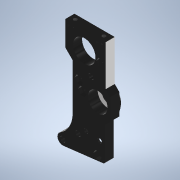
# Autodesk Inventor part: PartB_3gears_3D
Saved by Autodesk Inventor 2022 (Build 260153000, 153)
## iProperties
Created: 2020-12-02
Part Number: PartB_3gears_3D
Material: Generic
Document SubType Name: Modeling
Designer: Acer
Density: 1 g/cm^3
Appearance: Default
Author: Acer
Autodesk Inventor part; units mm, degrees
ref_plane "YZ Plane" through (0, 0, 0) normal (1, 0, 0) x (0, 1, 0)
ref_plane "XZ Plane" through (0, 0, 0) normal (0, 1, 0) x (-1, 0, 0)
ref_plane "XY Plane" through (0, 0, 0) normal (0, 0, 1) x (1, 0, 0)
sketch "Sketch1" plane through (0, 0, 0) normal (0, 0, 1) x (1, 0, 0)
  circle A0 centre (0, 0) radius 1.5
  circle A1 centre (0, 0) radius 3
  line L0 (0, 3) -> (23.5, 3)
  line L1 (23.5, 3) -> (23.5, -3)
  line L2 (23.5, -3) -> (0, -3)
  line L3 (0, -3) -> (0, 3)
  line L4 (23.5, 3) -> (5.5, 3)
  line L5 (5.5, 3) -> (5.5, 59)
  line L6 (5.5, 59) -> (23.5, 59)
  line L7 (23.5, 59) -> (23.5, 3)
  circle A2 centre (19.5, 27.75) radius 5.5
  circle A3 centre (11.9973, 48.75) radius 6.25
  line L8 (19.5, 27.75) -> (11.9973, 48.75) construction
  line L9 (19.5, 27.75) -> (5.5, 27.75) construction
  circle A4 centre (11.9973, 40.25) radius 1.05
  circle A5 centre (19.3585, 53) radius 1.05
  circle A6 centre (4.6361, 53) radius 1.05
  line L10 (5.5, 59) -> (1.5, 59)
  line L11 (1.5, 59) -> (1.5, 45)
  line L12 (1.5, 45) -> (5.5, 45)
  line L13 (5.5, 45) -> (5.5, 59)
  line L14 (1.5, 45) -> (5.5, 41)
  line L15 (1.5, 45) -> (7.1569, 45) construction
  line L16 (23.5, 33.75) -> (26.5, 33.75)
  line L17 (26.5, 33.75) -> (26.5, 21.75)
  line L18 (26.5, 21.75) -> (23.5, 21.75)
  line L19 (23.5, 21.75) -> (23.5, 33.75)
  line L20 (26.5, 33.75) -> (23.5, 36.75)
  line L21 (26.5, 33.75) -> (30.7426, 33.75) construction
  line L22 (26.5, 21.75) -> (23.5, 18.75)
  line L23 (26.5, 21.75) -> (30.7426, 21.75) construction
  circle A7 centre (8.5, 7) radius 1.5
  circle A8 centre (13, 10.5) radius 1.25
  circle A9 centre (20.5, 9.5) radius 1.25
  line L24 (11.9973, 48.75) -> (1.5, 48.75) construction
  line L25 (11.9973, 40.25) -> (11.9973, 48.75) construction
  circle A10 centre (15.7487, 38.25) radius 1.55
  circle A11 centre (11, 28.75) radius 1.05
  circle A12 centre (9, 33.25) radius 1.05
  circle A13 centre (21, 47.25) radius 1.05
  line L26 (5.5, 27) -> (23.5, 27) construction
  line L27 (23.5, 27) -> (23.5, 51) construction
  line L28 (23.5, 51) -> (5.5, 51) construction
  line L29 (5.5, 51) -> (5.5, 27) construction
  line L30 (7.7876, 31.15) -> (6.5751, 33.25) construction
  line L31 (6.5751, 33.25) -> (7.7876, 35.35) construction
  line L32 (7.7876, 35.35) -> (10.2124, 35.35) construction
  line L33 (10.2124, 35.35) -> (11.4249, 33.25) construction
  line L34 (11.4249, 33.25) -> (10.2124, 31.15) construction
  line L35 (10.2124, 31.15) -> (7.7876, 31.15) construction
  line L36 (9.7876, 26.65) -> (8.5751, 28.75) construction
  line L37 (8.5751, 28.75) -> (9.7876, 30.85) construction
  line L38 (9.7876, 30.85) -> (12.2124, 30.85) construction
  line L39 (12.2124, 30.85) -> (13.4249, 28.75) construction
  line L40 (13.4249, 28.75) -> (12.2124, 26.65) construction
  line L41 (12.2124, 26.65) -> (9.7876, 26.65) construction
  line L42 (23.5, -0.2) -> (0.1795, -3)
  dimension "d0" = 3
  dimension "d1" = 6
  dimension "d2" = 23.5
  dimension "d3" = 6
  dimension "d4" = 0
  dimension "d5" = 3
  dimension "d6" = 18
  dimension "d7" = 56
  dimension "d8" = 11
  dimension "d9" = 4
  dimension "d10" = 24.75
  dimension "d11" = 12.5
  dimension "d12" = 22.3
  dimension "d14" = 2.1
  dimension "d20" = 360
  dimension "d22" = 4
  dimension "d23" = 14
  dimension "d24" = 45
  dimension "d25" = 3
  dimension "d26" = 12
  dimension "d27" = 6
  dimension "d28" = 135
  dimension "d29" = 135
  dimension "d32" = 3
  dimension "d33" = 10
  dimension "d34" = 3
  dimension "d35" = 2.5
  dimension "d36" = 13.5
  dimension "d37" = 7.5
  dimension "d38" = 2.5
  dimension "d39" = 15
  dimension "d40" = 12.5
  dimension "d60" = 8.5
  dimension "d61" = 270
  dimension "d82" = 3.1
  dimension "d83" = 11.15
  dimension "d84" = 2.1
  dimension "d85" = 2.1
  dimension "d86" = 2.1
  dimension "d87" = 5.5
  dimension "d88" = 3.5
  dimension "d89" = 25.75
  dimension "d90" = 30.25
  dimension "d91" = 2.5
  dimension "d92" = 11.75
  dimension "d93" = 24
  dimension "d94" = 8
  dimension "d101" = 2.1
  dimension "d102" = 2.1
  dimension "d157" = 2.8
  constraints: 86 end point, 14 centre point, 11 horizontal, 10 parallel, 10 point on line, 6 perpendicular, 4 coincident, 3 equal length, 1 midpoint, 1 tangent, 33 other
  measures "d0" diameter of A0
  measures "d1" diameter of A1
  measures "d2" distance of L1.end L2.end
  measures "d3" distance of L0.end L1.end
  measures "d4" distance from line of point (0, 0) L3
  measures "d5" distance from line of L0 point (0, 0)
  measures "d6" distance of L5.end L6.end
  measures "d7" distance of L4.end L5.end
  measures "d8" diameter of A2
  measures "d9" distance from line of L7 L8.start
  measures "d10" distance from line of L8.start L0
  measures "d11" diameter of A3
  measures "d12" distance of L8.start L8.end
  measures "d14" diameter of A4
  measures "d22" distance of L12.end L11.end
  measures "d23" distance of L11.end L10.end
  measures "d24" angle of L14 L15
  measures "d25" distance of L17.end L18.end
  measures "d26" distance of L16.end L17.end
  measures "d27" distance from line of L16 L8.start
  measures "d28" angle of L21 L20
  measures "d29" angle of L22 L23
  measures "d32" diameter of A7
  measures "d33" distance from line of L2 A7.centre
  measures "d34" distance from line of L5 A7.centre
  measures "d35" diameter of A8
  measures "d36" distance from line of A8.centre L2
  measures "d37" distance from line of L5 A8.centre
  measures "d38" diameter of A9
  measures "d39" distance from line of A9.centre L5
  measures "d40" distance from line of L2 A9.centre
  measures "d60" distance of L25.start L8.end
  measures "d82" diameter of A10
  measures "d83" distance of A10.centre L8.start
  measures "d84" diameter of A11
  measures "d85" diameter of A12
  measures "d86" diameter of A13
  measures "d87" distance from line of L5 A11.centre
  measures "d88" distance from line of L5 A12.centre
  measures "d89" distance from line of L6 A12.centre
  measures "d90" distance from line of L6 A11.centre
  measures "d91" distance from line of L7 A13.centre
  measures "d92" distance from line of L6 A13.centre
  measures "d93" distance between parallel lines of L28 L26
  measures "d94" distance between parallel lines of L6 L28
  measures "d101" distance from line of A12.centre L35
  measures "d102" distance from line of A11.centre L41
  measures "d157" distance from line of L2 L42.start
extrude "Extrusion1" add sketch "Sketch1" along normal blind 5 contours A0 L3 A1 | A0 L3 A1 | L0 L1 L42 A1 | A1 L42 L2 | L5 A6 L6 L7 A2 L0 | L14 L12 L5 | L7 L18 L22 | L12 L11 L10 L5 A6 | L7 A2 L16 L17 L18 | A6 L5 | L5 A6 | L16 L7 L20 | A4 | A5
fillet "Fillet1" radius 1 1 edges at (23.5, -0.2, 2.5)
fillet "Fillet2" radius 15 1 edges at (5.5, 3, 2.5)
sketch "Sketch2" plane through (0, 0, 5) normal (0, 0, 1) x (1, 0, 0)
  line L0 (23.5, 0.6871) -> (23.5, 18.75) projected
  line L1 (0, -3) -> (0.1795, -3) projected
  line L2 (23.5, 0.6871) -> (23.5, 18.75) projected
  line L3 (23.5, 20.75) -> (10.75, 20.75)
  line L4 (10.75, 20.75) -> (10.75, 0.75)
  line L5 (10.75, 0.75) -> (23.5, 0.75)
  line L6 (23.5, 0.75) -> (23.5, 20.75)
  line L7 (23.5, 18.75) -> (26.5, 21.75) projected
  line L8 (23.5, 20.75) -> (25.5, 20.75)
  line L9 (23.5, 18.75) -> (26.5, 21.75) projected
  line L10 (22.25, 20.75) -> (22.25, 0.75)
  point P0 (0, 0)
  point P1 (23.5, -1)
  point P2 (21.5, -3)
  point P3 (23.5, 0.75)
  point P4 (23.5, 0.5)
  point P5 (23.5, 0.75)
  dimension "d43" = 12.75
  dimension "d44" = 20
  dimension "d45" = 23.75
  constraints: 12 end point, 4 point on line, 2 horizontal, 2 parallel, 2 perpendicular
  measures "d43" distance of L5.end L4.end
  measures "d44" distance of L4.end L3.end
  measures "d45" distance between parallel lines of L1 L3
extrude "Extrusion2" [suppressed]
sketch "Sketch3" plane through (1.5, 59, 0) normal (0, 1, 0) x (1, 0, 0)
  circle A0 centre (3, -2.5) radius 1
  line L0 (22, 0) -> (0, 0) projected
  line L1 (0, 0) -> (0, -5) projected
  line L2 (22, -5) -> (0, -5) projected
  line L3 (22, 0) -> (22, -5) projected
  circle A1 centre (19, -2.5) radius 1
  dimension "d48" = 2
  dimension "d49" = 2
  dimension "d50" = 2.5
  dimension "d51" = 2.5
  dimension "d52" = 3
  dimension "d53" = 3
  constraints: 2 centre point
  measures "d48" diameter of A0
  measures "d49" diameter of A1
  measures "d50" distance from line of L0 A0.centre
  measures "d51" distance from line of L0 A1.centre
  measures "d52" distance from line of A1.centre L3
  measures "d53" distance from line of L1 A0.centre
extrude "Extrusion3" cut sketch "Sketch3" against normal blind 4.5 contours A0 | A1
thread "Thread1" size "M2x0.4" class "6H" standard "ANSI Metric M Profile" length 7
thread "Thread2" size "M2x0.4" class "6H" standard "ANSI Metric M Profile" length 7
sketch "Sketch5" plane through (0, 0, 5) normal (0, 0, 1) x (1, 0, 0)
  circle A0 centre (11.9973, 40.25) radius 1.05 projected
  circle A1 centre (4.6361, 53) radius 1.05 projected
  circle A2 centre (19.3585, 53) radius 1.05 projected
  circle A3 centre (11.9973, 40.25) radius 2
  circle A4 centre (4.6361, 53) radius 2
  circle A5 centre (19.3585, 53) radius 2
  point P0 (0, 0)
  dimension "d62" = 4
  dimension "d63" = 4
  dimension "d64" = 4
  constraints: 3 centre point, 3 coincident
  measures "d62" diameter of A3
  measures "d63" diameter of A4
  measures "d64" diameter of A5
extrude "Extrusion4" [suppressed]
sketch "Sketch7" plane through (0, 0, 5) normal (0, 0, 1) x (1, 0, 0)
  circle A0 centre (8.5, 7) radius 1.5 projected
  circle A1 centre (8.5, 7) radius 2.75
  point P0 (0, 0)
  dimension "d67" = 5.5
  constraints: 1 centre point, 1 coincident
  measures "d67" diameter of A1
extrude "Extrusion5" cut sketch "Sketch7" against normal blind 2 contours A0 | A1
sketch "Sketch8" plane through (0, 0, 5) normal (0, 0, 1) x (1, 0, 0)
  line L0 (5.5, 59) -> (5.5, 54.5) projected
  line L1 (3.5, 59) -> (3.5, 54.5) projected
  circle A0 centre (19.5, 27.75) radius 5.5 projected
  circle A1 centre (11.9973, 48.75) radius 6.25 projected
  circle A2 centre (8.5, 7) radius 2.75 projected
  line L2 (23.5, 18.75) -> (26.5, 21.75) projected
  line L3 (26.5, 21.75) -> (26.5, 33.75) projected
  line L4 (26.5, 33.75) -> (23.5, 36.75) projected
  line L5 (23.5, 36.75) -> (23.5, 59) projected
  line L6 (23.5, 59) -> (1.5, 59) projected
  line L7 (1.5, 59) -> (1.5, 45) projected
  line L8 (1.5, 45) -> (5.5, 41) projected
  line L9 (5.5, 41) -> (5.5, 15.2889) projected
  line L10 (19.5, 59) -> (19.5, 54.5) projected
  line L11 (21.5, 59) -> (21.5, 54.5) projected
  line L12 (2.5, 55.275) -> (6.5, 55.275)
  line L13 (6.5, 55.275) -> (6.5, 57.125)
  line L14 (6.5, 57.125) -> (2.5, 57.125)
  line L15 (2.5, 57.125) -> (2.5, 55.275)
  line L16 (2.5, 55.275) -> (6.5, 57.125) construction
  line L17 (6.5, 55.275) -> (2.5, 57.125) construction
  line L18 (18.5, 57.125) -> (22.5, 57.125)
  line L19 (22.5, 57.125) -> (22.5, 55.275)
  line L20 (22.5, 55.275) -> (18.5, 55.275)
  line L21 (18.5, 55.275) -> (18.5, 57.125)
  line L22 (18.5, 57.125) -> (22.5, 55.275) construction
  line L23 (22.5, 57.125) -> (18.5, 55.275) construction
  arc A3 (-1.5833, 2.5481) -> (5.5, 15.2889) centre (-9.5, 15.2889) ccw projected
  arc A4 (-1.5833, 2.5481) -> (0, -3) centre (0, 0) ccw projected
  line L24 (0, -3) -> (0.1795, -3) projected
  line L25 (23.5, 0.6871) -> (23.5, 18.75) projected
  line L26 (0.1795, -3) -> (22.6192, -0.3058) projected
  arc A5 (22.6192, -0.3058) -> (23.5, 0.6871) centre (22.5, 0.6871) ccw projected
  point P0 (4.5, 56.2)
  point P1 (20.5, 56.2)
  dimension "d70" = 4
  dimension "d71" = 1.85
  dimension "d72" = 4
  dimension "d73" = 1.85
  dimension "d74" = 1
  dimension "d75" = 2.8
  dimension "d76" = 2.8
  dimension "d77" = 1
  constraints: 24 end point, 4 midpoint, 4 parallel, 2 horizontal, 2 perpendicular
  measures "d70" distance of L14.end L13.end
  measures "d71" distance of L13.end L12.end
  measures "d72" distance of L19.end L20.end
  measures "d73" distance of L18.end L19.end
  measures "d74" distance from line of point (4.5, 56.2) L0
  measures "d75" distance from line of L6 point (4.5, 56.2)
  measures "d76" distance from line of L6 point (20.5, 56.2)
  measures "d77" distance from line of point (20.5, 56.2) L11
extrude "Extrusion6" cut sketch "Sketch8" against normal up to surface (5 mm away) contours L14 L13 L12 L0 | L0 L12 L1 L14 | L1 L12 L15 L14 | L18 L11 L20 L10 | L10 L20 L21 L18 | L18 L19 L20 L11
sketch "Sketch10" plane through (0, 0, 0) normal (0, 0, -1) x (-1, 0, 0)
  circle A0 centre (-21, 47.25) radius 1.05 projected
  circle A1 centre (-9, 33.25) radius 1.05 projected
  circle A2 centre (-11, 28.75) radius 1.05 projected
  line L0 (-22.2124, 45.15) -> (-23.4249, 47.25)
  line L1 (-23.4249, 47.25) -> (-22.2124, 49.35)
  line L2 (-22.2124, 49.35) -> (-19.7876, 49.35)
  line L3 (-19.7876, 49.35) -> (-18.5751, 47.25)
  line L4 (-18.5751, 47.25) -> (-19.7876, 45.15)
  line L5 (-19.7876, 45.15) -> (-22.2124, 45.15)
  line L6 (-12.2124, 26.65) -> (-13.4249, 28.75)
  line L7 (-13.4249, 28.75) -> (-12.2124, 30.85)
  line L8 (-12.2124, 30.85) -> (-9.7876, 30.85)
  line L9 (-9.7876, 30.85) -> (-8.5751, 28.75)
  line L10 (-8.5751, 28.75) -> (-9.7876, 26.65)
  line L11 (-9.7876, 26.65) -> (-12.2124, 26.65)
  line L12 (-10.2124, 31.15) -> (-11.4249, 33.25)
  line L13 (-11.4249, 33.25) -> (-10.2124, 35.35)
  line L14 (-10.2124, 35.35) -> (-7.7876, 35.35)
  line L15 (-7.7876, 35.35) -> (-6.5751, 33.25)
  line L16 (-6.5751, 33.25) -> (-7.7876, 31.15)
  line L17 (-7.7876, 31.15) -> (-10.2124, 31.15)
  point P0 (0, 0)
  point P1 (-13.9053, 32.1)
  point P2 (-12.0947, 30.9)
  dimension "d95" = 2.1
  dimension "d96" = 2.1
  dimension "d98" = 2.1
  constraints: 36 end point, 4 coincident, 3 horizontal, 39 other
  measures "d95" distance from line of A0.centre L5
  measures "d96" distance from line of A2.centre L11
  measures "d98" distance from line of A1.centre L17
extrude "Extrusion7" cut sketch "Sketch10" against normal blind 1.8 contours A1 | A2 | L0 L1 L2 L3 L4 L5 | L6 L7 L8 L9 L10 L11 | L12 L13 L14 L15 L16 L17
sketch "Sketch13" plane through (0, 0, 0) normal (0, 0, -1) x (-1, 0, 0)
  circle A0 centre (-13, 10.5) radius 1.25 projected
  line L0 (-10.5751, 10.5) -> (-11.7876, 8.4)
  line L1 (-11.7876, 8.4) -> (-14.2124, 8.4)
  line L2 (-14.2124, 8.4) -> (-15.4249, 10.5)
  line L3 (-15.4249, 10.5) -> (-14.2124, 12.6)
  line L4 (-14.2124, 12.6) -> (-11.7876, 12.6)
  line L5 (-11.7876, 12.6) -> (-10.5751, 10.5)
  point P0 (0, 0)
  dimension "d103" = 2.1
  constraints: 12 end point, 1 coincident, 13 other
  measures "d103" distance from line of L1 point (-13, 10.5)
extrude "Extrusion8" [suppressed]
sketch "Sketch15" plane through (0, 0, 5) normal (0, 0, 1) x (1, 0, 0)
  line L0 (23.5, 0.6871) -> (23.5, 18.75) projected
  line L1 (23.5, 18.75) -> (26.5, 21.75) projected
  line L2 (0, -3) -> (0.1795, -3) projected
  circle A0 centre (20.5, 9.5) radius 1.25 projected
  line L3 (15.75, 19.5) -> (23, 19.5)
  line L4 (23, 19.5) -> (23, 4.5)
  line L5 (23, 4.5) -> (15.75, 4.5)
  line L6 (15.75, 4.5) -> (15.75, 19.5)
  line L7 (15.75, 14.5) -> (10.75, 14.5)
  line L8 (10.75, 14.5) -> (10.75, 9.5)
  line L9 (10.75, 9.5) -> (15.75, 9.5)
  line L10 (15.75, 9.5) -> (15.75, 14.5)
  line L11 (15.75, 4.5) -> (10.75, 9.5)
  line L12 (10.75, 14.5) -> (15.75, 19.5)
  line L13 (10.75, 14.5) -> (5.5, 19.75)
  line L14 (5.5, 41) -> (5.5, 15.2889) projected
  line L15 (15.75, 19.5) -> (5.5, 29.75)
  point P0 (0, 0)
  point P1 (0, 0)
  point P2 (23.5, -1)
  point P3 (21.5, -3)
  point P4 (23.5, 0.5)
  dimension "d125" = 5
  dimension "d126" = 7.25
  dimension "d127" = 2.5
  dimension "d128" = 5
  dimension "d129" = 15
  dimension "d130" = 5
  dimension "d131" = 5
  dimension "d132" = 90
  dimension "d133" = 135
  constraints: 24 end point, 4 parallel, 3 point on line, 2 horizontal, 2 perpendicular
  measures "d125" distance from line of A0.centre L5
  measures "d126" distance of L4.end L5.end
  measures "d127" distance from line of A0.centre L4
  measures "d128" distance between parallel lines of L6 L8
  measures "d129" distance of L5.end L3.start
  measures "d130" distance from line of L5.end L9
  measures "d131" distance from line of L3.start L7
  measures "d132" angle of L13 L12
  measures "d133" angle of L3 L15
extrude "Extrusion9" cut sketch "Sketch15" against normal blind 3.9 contours L3 L4 L5 L6 | L6 L7 L12 | L6 L9 L8 L7 | L6 L11 L9
sketch "Sketch17" plane through (0, 0, 0) normal (0, 0, -1) x (-1, 0, 0)
  line L0 (-26.5, 21.75) -> (-26.5, 3.75)
  line L1 (-26.5, 3.75) -> (-23.5, 3.75)
  line L2 (-23.5, 0.6871) -> (-23.5, 18.75) projected
  line L3 (-23.5, 3.75) -> (-23.5, 18.75)
  line L4 (-23.5, 20.7) -> (-23.5, 18.75) projected
  line L5 (-23.5, 18.75) -> (-26.5, 18.75)
  line L6 (-26.5, 21.75) -> (-23.5, 18.75)
  point P0 (0, 0)
  point P1 (-23.5, -1)
  point P2 (-23.5, 3.75)
  point P3 (-23.5, 0.5)
  dimension "d119" = 18
  constraints: 10 end point, 3 perpendicular, 1 point on line, 1 vertical
  measures "d119" distance of L0.start L0.end
extrude "Extrusion10" [suppressed]
fillet "Fillet3" [suppressed]
sketch "Sketch19" plane through (0, 0, 5) normal (0, 0, 1) x (1, 0, 0)
  circle A0 centre (13, 10.5) radius 1.25 projected
  line L0 (10.75, 9.5) -> (10.75, 14.5) projected
  line L1 (15.75, 4.5) -> (10.75, 9.5) projected
  line L2 (23, 4.5) -> (15.75, 4.5) projected
  line L3 (23, 19.5) -> (23, 4.5) projected
  line L4 (15.75, 19.5) -> (23, 19.5) projected
  line L5 (10.75, 14.5) -> (15.75, 19.5) projected
  circle A1 centre (20.5, 9.5) radius 1.25 projected
  line L6 (10.75, 9.5) -> (10.75, 14.5) projected
  line L7 (5.5, 41) -> (5.5, 15.2889) projected
  line L8 (10.75, 14.5) -> (15.75, 19.5) projected
  line L9 (10.75, 14.5) -> (5.5, 19.75)
  line L10 (5.5, 41) -> (5.5, 15.2889) projected
  line L11 (10.75, 14.5) -> (18.1746, 14.5) construction
  line L12 (15.75, 19.5) -> (5.5, 29.75)
  line L13 (15.75, 19.5) -> (30.2457, 19.5) construction
  point P0 (0, 0)
  dimension "d135" = 135
  dimension "d136" = 135
  constraints: 8 end point, 2 equal length, 2 horizontal, 2 point on line
  measures "d135" angle of L11 L9
  measures "d136" angle of L13 L12
extrude "Extrusion11" cut sketch "Sketch19" against normal blind 3 contours L9 L7 L12 L5
chamfer "Chamfer1" distance 0.9 angle 45 1 edges at (13.25, 17, 2)
fillet "Fillet4" radius 4 1 edges at (12.6137, 17.6363, 2)
sketch "Sketch21" plane through (0, 0, 5) normal (0, 0, 1) x (1, 0, 0)
  circle A0 centre (19.375, 1.9) radius 1
  circle A1 centre (13, 10.5) radius 1.25 projected
  line L0 (10.75, 9.5) -> (10.75, 14.5) projected
  line L1 (15.75, 4.5) -> (10.75, 9.5) projected
  line L2 (23, 4.5) -> (15.75, 4.5) projected
  line L3 (23, 19.5) -> (23, 4.5) projected
  line L4 (15.75, 19.5) -> (23, 19.5) projected
  line L5 (10.75, 14.5) -> (15.75, 19.5) projected
  circle A2 centre (20.5, 9.5) radius 1.25 projected
  point P0 (0, 0)
  dimension "d143" = 2
  dimension "d144" = 2.6
  dimension "d145" = 3.625
  constraints: 1 centre point
  measures "d143" diameter of A0
  measures "d144" distance from line of L2 A0.centre
  measures "d145" distance from line of A0.centre L3
extrude "Extrusion12" cut sketch "Sketch21" against normal up to surface (5 mm away) contours A0
sketch "Sketch22" plane through (0, 0, 0) normal (0, 0, -1) x (-1, 0, 0)
  circle A0 centre (-19.375, 1.9) radius 1 projected
  line L0 (-20.5586, -0.15) -> (-21.7421, 1.9)
  line L1 (-21.7421, 1.9) -> (-20.5586, 3.95)
  line L2 (-20.5586, 3.95) -> (-18.1914, 3.95)
  line L3 (-18.1914, 3.95) -> (-17.0079, 1.9)
  line L4 (-17.0079, 1.9) -> (-18.1914, -0.15)
  line L5 (-18.1914, -0.15) -> (-20.5586, -0.15)
  point P0 (0, 0)
  dimension "d148" = 2.05
  constraints: 12 end point, 1 coincident, 1 horizontal, 13 other
  measures "d148" distance from line of A0.centre L5
extrude "Extrusion13" cut sketch "Sketch22" against normal blind 2.4 contours A0 | L0 L1 L2 L3 L4 L5
sketch "Sketch23" plane through (0, 0, 5) normal (0, 0, 1) x (1, 0, 0)
  circle A0 centre (13, 10.5) radius 1.25 projected
  line L0 (10.75, 9.5) -> (10.75, 14.5) projected
  line L1 (15.75, 4.5) -> (10.75, 9.5) projected
  line L2 (23, 4.5) -> (15.75, 4.5) projected
  line L3 (23, 19.5) -> (23, 4.5) projected
  line L4 (15.75, 19.5) -> (23, 19.5) projected
  line L5 (10.75, 14.5) -> (15.75, 19.5) projected
  circle A1 centre (20.5, 9.5) radius 1.25 projected
  line L6 (23, 4.5) -> (15.75, 4.5)
  line L7 (15.75, 4.5) -> (15.75, 0)
  line L8 (15.75, 0) -> (23, 0)
  line L9 (23, 0) -> (23, 4.5)
  point P0 (0, 0)
  dimension "d151" = 4.5
  constraints: 8 end point, 2 parallel, 1 horizontal, 1 perpendicular
  measures "d151" distance between parallel lines of L2 L8
extrude "Extrusion14" cut sketch "Sketch23" against normal blind 1 contours L2 L9 L8 L7
fillet "Fillet5" radius 2 2 edges at (15.75, 0, 4.5) (23, 0, 4.5)
mirror "Mirror2" about plane through (11.75, 28, 0) normal (0, 0, -1) remove original yes
sketch "Sketch24" plane through (23.5, 59, -5) normal (0, 0, -1) x (-1, 0, 0)
  circle A0 centre (4, -31.25) radius 5.5 projected
  circle A1 centre (4, -31.25) radius 6.5
  circle A2 centre (4, -31.25) radius 3
  point P0 (23.5, -59)
  dimension "d158" = 1
  dimension "d164" = 6
  constraints: 2 centre point, 1 coincident
  measures "d158" radial gap between concentric circles of A0 A1
  measures "d164" diameter of A2
extrude "Extrusion15" add sketch "Sketch24" along normal blind 1.5 contours A0 | A1
chamfer "Chamfer2" distance 1.5 angle 45 1 edges at (26, 27.75, -5)
sketch "Sketch25" plane through (1.5, 59, 0) normal (0, 0, 1) x (1, 0, 0)
  line L0 (22, -22.25) -> (22, 0) projected
  line L1 (22.5, -22.75) -> (22.5, 0)
  line L2 (25, -25.25) -> (22, -22.25) projected
  line L3 (22, 0) -> (0, 0) projected
  line L4 (22, 0) -> (22.5, 0)
  point P0 (-1.5, -59)
  dimension "d165" = 0.5
  constraints: 4 end point, 1 collinear, 1 parallel, 1 point on line
  measures "d165" distance between parallel lines of L0 L1
extrude "Extrusion16" add sketch "Sketch25" against normal up to surface (5 mm away)
sketch "Sketch26" plane through (19.5, 27.75, -5) normal (0, 0, 1) x (1, 0, 0)
  circle A0 centre (0, 0) radius 5.5 projected
  point P0 (-19.5, -27.75)
extrude "Extrusion17" cut sketch "Sketch26" against normal blind 0.5
body "Solid1"
